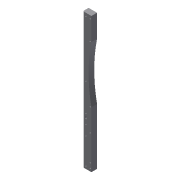
# Autodesk Inventor part: Claw - Arm - Top (R) Bottom
Saved by Autodesk Inventor 2015 (Build 190159000, 159)
## iProperties
Created: 2015-01-10
Part Number: Claw - Arm - Top (R) Bottom
Material: Generic
Document SubType Name: Sheet Metal
Designer: Tanner
Density: 1 g/cm^3
Sheet Metal Rule: Default
Appearance: Default
Flat Pattern Width: 60.8635 cm
Flat Pattern Length: 3.81 cm
Flat Pattern Area: 231.89 cm^2
Sheet Metal Width: 23.962 in
Sheet Metal Length: 1.500 in
Sheet Metal Area: 35.943 in^2
Author: Tanner
Autodesk Inventor part; units mm, degrees
ref_plane "YZ Plane" through (0, 0, 0) normal (1, 0, 0) x (0, 1, 0)
ref_plane "XZ Plane" through (0, 0, 0) normal (0, 1, 0) x (-1, 0, 0)
ref_plane "XY Plane" through (0, 0, 0) normal (0, 0, 1) x (1, 0, 0)
sketch "Sketch1" plane through (0, 0, 0) normal (0, 0, 1) x (1, 0, 0)
  line L0 (0, 0) -> (38.1, 0)
  line L1 (38.1, 0) -> (38.1, 253.0348)
  arc A0 (38.1, 507.0348) -> (38.1, 253.0348) centre (666.75, 380.0348) ccw
  line L2 (38.1, 507.0348) -> (38.1, 608.6348)
  line L3 (38.1, 608.6348) -> (0, 608.6348)
  line L4 (0, 608.6348) -> (0, 0)
  circle A1 centre (31.75, 151.4348) radius 3.3655
  circle A2 centre (31.75, 34.671) radius 3.3655
  circle A3 centre (12.7, 12.7) radius 3.3655
  circle A4 centre (12.7, 342.9) radius 3.3655
  circle A5 centre (12.7, 595.9348) radius 3.3655
  circle A6 centre (31.75, 12.7) radius 3.3655
  circle A7 centre (31.75, 253.0348) radius 3.3655
  circle A8 centre (31.75, 507.0348) radius 3.3655
  circle A9 centre (31.75, 595.9348) radius 3.3655
  line L5 (0, 557.8348) -> (0, 608.6348)
  line L6 (0, 50.8) -> (0, 0)
  line L7 (12.7, 342.9) -> (0, 304.3174) construction
  line L8 (0, 317.5) -> (0, 368.3)
  line L9 (0, 129.921) -> (12.7, 129.921) construction
  circle A10 centre (12.7, 129.921) radius 3.3655
  circle A11 centre (12.7, 174.371) radius 3.3655
  line L10 (9.3413, 197.482) -> (9.3413, 204.213)
  line L11 (16.0611, 204.488) -> (16.0611, 197.3435)
  arc A12 (16.0611, 204.488) -> (9.3413, 204.213) centre (12.6956, 204.488) ccw
  arc A13 (9.3413, 197.482) -> (16.0611, 197.3435) centre (12.6974, 197.231) ccw
  circle A14 centre (12.7, 217.188) radius 3.3655
  dimension "d0" = 38.1
  dimension "d2" = 101.6
  dimension "d4" = 457.2
  dimension "d5" = 101.6
  dimension "d6" = 666.75
  dimension "d7" = 641.35
  dimension "d9" = 116.7638
  dimension "d10" = 6.35
  dimension "d11" = 6.35
  dimension "d13" = 12.7
  dimension "d14" = 12.7
  dimension "d16" = 12.7
  dimension "d17" = 342.9
  dimension "d19" = 12.7
  dimension "d20" = 12.7
  dimension "d22" = 6.35
  dimension "d24" = 6.35
  dimension "d25" = 6.731
  dimension "d26" = 6.35
  dimension "hole" = 6.731
  dimension "d28" = 6.35
  dimension "d45" = 12.7
  dimension "d47" = 12.7
  dimension "d54" = 6.731
  dimension "d55" = 3.3655
  dimension "d56" = 3.3655
  dimension "d58" = 6.731
  dimension "d59" = 12.7
  dimension "d68" = 18.22
  dimension "d69" = 90
  dimension "d70" = 90
  dimension "d71" = 22.0389
  dimension "d72" = 28.7587
  dimension "d73" = 478.7138
  dimension "d74" = 6.35
  dimension "d75" = 6.35
  dimension "d76" = 595.9348
  dimension "d77" = 404.1468
  dimension "d78" = 411.2913
  dimension "d79" = 25.4
  dimension "d80" = 25.4
  dimension "d81" = 434.2638
  dimension "d82" = 50.8
  dimension "d83" = 240.3348
  dimension "d84" = 291.1348
  dimension "d85" = 557.8348
  constraints: 24 end point, 15 centre point, 9 equal radius, 6 point on circle, 4 perpendicular, 3 parallel, 2 point on line, 1 coincident, 1 collinear, 1 horizontal, 1 midpoint, 1 tangent, 1 vertical
  measures "d0" distance of L2.end L3.end
  measures "d2" distance of L2.start L2.end
  measures "d4" distance from line of A1.centre L3
  measures "d5" vertical distance of L1.end A1.centre
  measures "d6" distance from line of A0.centre L4
  measures "d7" radius of A0
  measures "d9" distance of A1.centre A2.centre
  measures "d10" distance from line of L1 A2.centre
  measures "d11" distance from line of A1.centre L1
  measures "d13" distance from line of A3.centre L0
  measures "d14" distance from line of L4 A3.centre
  measures "d16" distance from line of L4 L7.start
  measures "d17" distance from line of L7.start L0
  measures "d19" distance from line of L3 A5.centre
  measures "d20" distance from line of L4 A5.centre
  measures "d22" distance from line of L1 A6.centre
  measures "d24" distance of L1.end A7.centre
  measures "d25" diameter of A8
  measures "d26" distance of L2.start A8.centre
  measures "hole" diameter of A9
  measures "d28" distance from line of L2 A9.centre
  measures "d45" distance from line of A9.centre L3
  measures "d47" distance of L9.start L9.end
  measures "d54" distance of L10.start L10.end
  measures "d55" radius of A12
  measures "d56" radius of A13
  measures "d58" diameter of A14
  measures "d59" distance of A12.centre A14.centre
  measures "d68" angle of L7 L1
  measures "d69" angle of L5 L3
  measures "d70" angle of L8 L3
  measures "d71" distance between parallel lines of L1 L11
  measures "d72" distance between parallel lines of L1 L10
  measures "d73" distance between parallel lines of L9 L3
  measures "d74" distance from line of A8.centre L1
  measures "d75" distance from line of A7.centre L1
  measures "d76" distance from line of A6.centre L3
  measures "d77" distance from line of L11.start L3
  measures "d78" distance from line of L11.end L3
  measures "d79" distance from line of A14.centre L1
  measures "d80" distance from line of A11.centre L1
  measures "d81" distance from line of A11.centre L3
  measures "d82" distance from line of L5.start L3
  measures "d83" distance from line of L8.end L3
  measures "d84" distance from line of L8.start L3
  measures "d85" distance from line of L6.start L3
extrude "Extrusion2" add sketch "Sketch1" along normal blind 25.4
fillet "Fillet1" radius 6.096 2 edges at (0, 184.15, 25.4) (0, 488.4674, 25.4)
equation "\"d25\" = hole"
equation "\"BendRadius\" = Thickness"
equation "\"BendReliefWidth\" = Thickness"
equation "\"BendReliefDepth\" = 0.5 * Thickness"
equation "\"CornerReliefSize\" = 4 * Thickness"
equation "\"MinimumRemnant\" = 2 * Thickness"
equation "\"TransitionRadius\" = BendRadius"
equation "\"JacobiRadiusSize\" = BendRadius"
equation "\"GapSize\" = Thickness"
equation "\"d29\" = BendRadius"
equation "\"d32\" = BendRadius"
equation "\"d38\" = BendRadius"
equation "\"d60\" = BendRadius"
equation "\"Thickness\" = 3.048"
body "Solid4"
